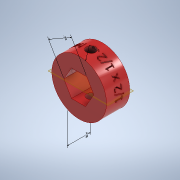
# Autodesk Inventor part: 1_2x1_2-hexBearingSplitA
Saved by Autodesk Inventor 2022.1 (Build 261234000, 234)
## iProperties
Created: 2020-11-08
Part Number: 1_2x1_2-hexBearingSplitA
Material: PC/ABS Plastic
Document SubType Name: Modeling
Designer: robst
Density: 0.357273 g/cm^3
Appearance: Red
Author: robst
Autodesk Inventor part; units mm, degrees
ref_plane "YZ Plane" through (0, 0, 0) normal (1, 0, 0) x (0, 1, 0)
ref_plane "XY Plane" through (0, 0, 0) normal (0, 0, 1) x (1, 0, 0)
sketch "Sketch1" plane through (0, 0, 0) normal (0, 0, 1) x (1, 0, 0)
  line L0 (3.6662, 6.35) -> (7.3323, 0)
  line L1 (7.3323, 0) -> (3.6662, -6.35)
  line L2 (3.6662, -6.35) -> (-3.6662, -6.35)
  line L3 (-3.6662, -6.35) -> (-7.3323, 0)
  line L4 (-7.3323, 0) -> (-3.6662, 6.35)
  line L5 (-3.6662, 6.35) -> (3.6662, 6.35)
  circle A0 centre (0, 0) radius 14.2875
  circle A1 centre (0, 0) radius 7.3323 construction
  dimension "d0" = 12.7
  dimension "d2" = 28.575
  dimension "d3" = 6.9551
  constraints: 12 end point, 3 coincident, 1 centre point, 1 horizontal, 1 horizontal alignment, 15 other
  measures "d0" distance between parallel lines of L2 L5
  measures "d2" diameter of A0
extrude "Extrusion1" add sketch "Sketch1" against normal blind 12.7
thicken "Thicken2" operation add thickness 0.5715 both sides no extend neighbours yes toward (-0.8660254, -0.5, 0) faces at (-4.8882, -4.2333, -4.2333) (-6.1103, 2.1167, -4.2333) (-1.2221, 6.35, -4.2333) (4.8882, 4.2333, -4.2333) (7.8832, 4.3299, 0) (1.2221, -6.35, -4.2333)
ref_plane "Work Plane1" through (0, 14.2875, 0) normal (0, 1, 0) x (-1, 0, 0)
sketch "Sketch2" plane through (0, 14.2875, 0) normal (0, 1, 0) x (-1, 0, 0)
  line L0 (0, -6.9215) -> (-25.4, -6.9215) construction
  line L1 (14.2875, -0.5715) -> (-14.2875, -0.5715) construction
  line L2 (-22.9639, -8.8265) -> (-24.8226, -8.8265)
  line L3 (-24.8226, -8.8265) -> (-24.8226, -8.4375)
  line L4 (-24.8226, -8.4375) -> (-24.131, -8.4375)
  line L5 (-24.131, -8.4375) -> (-24.131, -5.8841)
  line L6 (-24.131, -5.8841) -> (-24.8226, -5.8841)
  line L7 (-24.8226, -5.8841) -> (-24.8226, -5.5352)
  spline S0 degree 2 poles (-24.8226, -5.5352) (-24.4305, -5.5352) (-24.06, -5.3129) (-24.0353, -5.0041) knots 0 0 0 1 2 2 2
  line L8 (-24.0353, -5.0041) -> (-23.6401, -5.0041)
  line L9 (-23.6401, -5.0041) -> (-23.6401, -8.4375)
  line L10 (-23.6401, -8.4375) -> (-22.9639, -8.4375)
  line L11 (-22.9639, -8.4375) -> (-22.9639, -8.8265)
  line L12 (-20.6792, -4.8467) -> (-22.1705, -9.654)
  line L13 (-22.1705, -9.654) -> (-22.6027, -9.654)
  line L14 (-22.6027, -9.654) -> (-21.1176, -4.8467)
  line L15 (-21.1176, -4.8467) -> (-20.6792, -4.8467)
  line L16 (-17.9097, -8.8265) -> (-20.2593, -8.8265)
  line L17 (-20.2593, -8.8265) -> (-20.2593, -8.2862)
  spline S1 degree 2 poles (-20.2593, -8.2862) (-20.0061, -8.0484) (-19.5553, -7.6069) (-19.3392, -7.3692) knots 0 0 0 1 2 2 2
  spline S2 degree 2 poles (-19.3392, -7.3692) (-18.9039, -6.8906) (-18.5858, -6.3163) (-18.5858, -6.0107) knots 0 0 0 1 2 2 2
  spline S3 degree 2 poles (-18.5858, -6.0107) (-18.5858, -5.8501) (-18.6846, -5.6093) (-18.7742, -5.5321) knots 0 0 0 1 2 2 2
  spline S4 degree 2 poles (-18.7742, -5.5321) (-18.8637, -5.4549) (-19.0984, -5.3777) (-19.2404, -5.3777) knots 0 0 0 1 2 2 2
  spline S5 degree 2 poles (-19.2404, -5.3777) (-19.3762, -5.3777) (-19.6541, -5.4457) (-19.7807, -5.4982) knots 0 0 0 1 2 2 2
  spline S6 degree 2 poles (-19.7807, -5.4982) (-19.8888, -5.5414) (-20.0895, -5.6649) (-20.1512, -5.7081) knots 0 0 0 1 2 2 2
  line L18 (-20.1512, -5.7081) -> (-20.179, -5.7081)
  line L19 (-20.179, -5.7081) -> (-20.179, -5.1647)
  spline S7 degree 2 poles (-20.179, -5.1647) (-20.0215, -5.0875) (-19.4565, -4.9362) (-19.2033, -4.9362) knots 0 0 0 1 2 2 2
  spline S8 degree 2 poles (-19.2033, -4.9362) (-18.6692, -4.9362) (-18.0671, -5.5012) (-18.0671, -5.9829) knots 0 0 0 1 2 2 2
  spline S9 degree 2 poles (-18.0671, -5.9829) (-18.0671, -6.2083) (-18.1721, -6.585) (-18.2647, -6.7455) knots 0 0 0 1 2 2 2
  spline S10 degree 2 poles (-18.2647, -6.7455) (-18.3574, -6.9122) (-18.626, -7.2395) (-18.7742, -7.397) knots 0 0 0 1 2 2 2
  spline S11 degree 2 poles (-18.7742, -7.397) (-19.015, -7.6594) (-19.6047, -8.2213) (-19.7807, -8.385) knots 0 0 0 1 2 2 2
  line L20 (-19.7807, -8.385) -> (-17.9097, -8.385)
  line L21 (-17.9097, -8.385) -> (-17.9097, -8.8265)
  line L22 (-13.4729, -8.8265) -> (-14.0626, -8.8265)
  line L23 (-14.0626, -8.8265) -> (-14.7573, -7.752)
  line L24 (-14.7573, -7.752) -> (-15.4705, -8.8265)
  line L25 (-15.4705, -8.8265) -> (-16.017, -8.8265)
  line L26 (-16.017, -8.8265) -> (-15.0259, -7.4093)
  line L27 (-15.0259, -7.4093) -> (-16.0078, -5.9675)
  line L28 (-16.0078, -5.9675) -> (-15.418, -5.9675)
  line L29 (-15.418, -5.9675) -> (-14.7264, -7.0327)
  line L30 (-14.7264, -7.0327) -> (-14.0194, -5.9675)
  line L31 (-14.0194, -5.9675) -> (-13.4729, -5.9675)
  line L32 (-13.4729, -5.9675) -> (-14.4578, -7.3785)
  line L33 (-14.4578, -7.3785) -> (-13.4729, -8.8265)
  line L34 (-9.3758, -8.8265) -> (-11.2345, -8.8265)
  line L35 (-11.2345, -8.8265) -> (-11.2345, -8.4375)
  line L36 (-11.2345, -8.4375) -> (-10.5429, -8.4375)
  line L37 (-10.5429, -8.4375) -> (-10.5429, -5.8841)
  line L38 (-10.5429, -5.8841) -> (-11.2345, -5.8841)
  line L39 (-11.2345, -5.8841) -> (-11.2345, -5.5352)
  spline S12 degree 2 poles (-11.2345, -5.5352) (-10.8423, -5.5352) (-10.4718, -5.3129) (-10.4471, -5.0041) knots 0 0 0 1 2 2 2
  line L40 (-10.4471, -5.0041) -> (-10.0519, -5.0041)
  line L41 (-10.0519, -5.0041) -> (-10.0519, -8.4375)
  line L42 (-10.0519, -8.4375) -> (-9.3758, -8.4375)
  line L43 (-9.3758, -8.4375) -> (-9.3758, -8.8265)
  line L44 (-7.091, -4.8467) -> (-8.5823, -9.654)
  line L45 (-8.5823, -9.654) -> (-9.0145, -9.654)
  line L46 (-9.0145, -9.654) -> (-7.5294, -4.8467)
  line L47 (-7.5294, -4.8467) -> (-7.091, -4.8467)
  line L48 (-4.3215, -8.8265) -> (-6.6711, -8.8265)
  line L49 (-6.6711, -8.8265) -> (-6.6711, -8.2862)
  spline S13 degree 2 poles (-6.6711, -8.2862) (-6.4179, -8.0484) (-5.9671, -7.6069) (-5.751, -7.3692) knots 0 0 0 1 2 2 2
  spline S14 degree 2 poles (-5.751, -7.3692) (-5.3157, -6.8906) (-4.9977, -6.3163) (-4.9977, -6.0107) knots 0 0 0 1 2 2 2
  spline S15 degree 2 poles (-4.9977, -6.0107) (-4.9977, -5.8501) (-5.0965, -5.6093) (-5.186, -5.5321) knots 0 0 0 1 2 2 2
  spline S16 degree 2 poles (-5.186, -5.5321) (-5.2755, -5.4549) (-5.5102, -5.3777) (-5.6522, -5.3777) knots 0 0 0 1 2 2 2
  spline S17 degree 2 poles (-5.6522, -5.3777) (-5.7881, -5.3777) (-6.0659, -5.4457) (-6.1925, -5.4982) knots 0 0 0 1 2 2 2
  spline S18 degree 2 poles (-6.1925, -5.4982) (-6.3006, -5.5414) (-6.5013, -5.6649) (-6.563, -5.7081) knots 0 0 0 1 2 2 2
  line L50 (-6.563, -5.7081) -> (-6.5908, -5.7081)
  line L51 (-6.5908, -5.7081) -> (-6.5908, -5.1647)
  spline S19 degree 2 poles (-6.5908, -5.1647) (-6.4334, -5.0875) (-5.8683, -4.9362) (-5.6152, -4.9362) knots 0 0 0 1 2 2 2
  spline S20 degree 2 poles (-5.6152, -4.9362) (-5.081, -4.9362) (-4.479, -5.5012) (-4.479, -5.9829) knots 0 0 0 1 2 2 2
  spline S21 degree 2 poles (-4.479, -5.9829) (-4.479, -6.2083) (-4.5839, -6.585) (-4.6766, -6.7455) knots 0 0 0 1 2 2 2
  spline S22 degree 2 poles (-4.6766, -6.7455) (-4.7692, -6.9122) (-5.0378, -7.2395) (-5.186, -7.397) knots 0 0 0 1 2 2 2
  spline S23 degree 2 poles (-5.186, -7.397) (-5.4268, -7.6594) (-6.0165, -8.2213) (-6.1925, -8.385) knots 0 0 0 1 2 2 2
  line L52 (-6.1925, -8.385) -> (-4.3215, -8.385)
  line L53 (-4.3215, -8.385) -> (-4.3215, -8.8265)
  line L54 (6.6855, -8.8265) -> (6.2039, -8.8265)
  line L55 (6.2039, -8.8265) -> (6.2039, -7.1963)
  spline S24 degree 2 poles (6.2039, -7.1963) (6.2039, -6.9987) (6.1668, -6.6591) (6.1112, -6.5572) knots 0 0 0 1 2 2 2
  spline S25 degree 2 poles (6.1112, -6.5572) (6.0526, -6.4491) (5.8426, -6.3441) (5.6635, -6.3441) knots 0 0 0 1 2 2 2
  spline S26 degree 2 poles (5.6635, -6.3441) (5.4845, -6.3441) (5.1047, -6.5356) (4.9225, -6.6899) knots 0 0 0 1 2 2 2
  line L56 (4.9225, -6.6899) -> (4.9225, -8.8265)
  line L57 (4.9225, -8.8265) -> (4.4409, -8.8265)
  line L58 (4.4409, -8.8265) -> (4.4409, -4.8467)
  line L59 (4.4409, -4.8467) -> (4.9225, -4.8467)
  line L60 (4.9225, -4.8467) -> (4.9225, -6.2855)
  spline S27 degree 2 poles (4.9225, -6.2855) (5.1387, -6.091) (5.5555, -5.8872) (5.7901, -5.8872) knots 0 0 0 1 2 2 2
  spline S28 degree 2 poles (5.7901, -5.8872) (6.21, -5.8872) (6.6855, -6.4429) (6.6855, -6.9709) knots 0 0 0 1 2 2 2
  line L61 (6.6855, -6.9709) -> (6.6855, -8.8265)
  spline S29 degree 2 poles (8.6029, -8.8913) (7.9174, -8.8913) (7.1641, -8.1225) (7.1641, -7.4124) knots 0 0 0 1 2 2 2
  spline S30 degree 2 poles (7.1641, -7.4124) (7.1641, -6.7146) (7.8958, -5.8872) (8.4855, -5.8872) knots 0 0 0 1 2 2 2
  spline S31 degree 2 poles (8.4855, -5.8872) (8.7511, -5.8872) (9.1617, -6.0416) (9.313, -6.2052) knots 0 0 0 1 2 2 2
  spline S32 degree 2 poles (9.313, -6.2052) (9.4674, -6.3688) (9.631, -6.8412) (9.631, -7.1839) knots 0 0 0 1 2 2 2
  line L62 (9.631, -7.1839) -> (9.631, -7.4464)
  line L63 (9.631, -7.4464) -> (7.6519, -7.4464)
  spline S33 degree 2 poles (7.6519, -7.4464) (7.6519, -7.9435) (8.1521, -8.4714) (8.5967, -8.4714) knots 0 0 0 1 2 2 2
  spline S34 degree 2 poles (8.5967, -8.4714) (8.7541, -8.4714) (9.0598, -8.4004) (9.1833, -8.3448) knots 0 0 0 1 2 2 2
  spline S35 degree 2 poles (9.1833, -8.3448) (9.313, -8.2831) (9.4921, -8.175) (9.5507, -8.1256) knots 0 0 0 1 2 2 2
  line L64 (9.5507, -8.1256) -> (9.5785, -8.1256)
  line L65 (9.5785, -8.1256) -> (9.5785, -8.6505)
  spline S36 degree 2 poles (9.5785, -8.6505) (9.4952, -8.6845) (9.242, -8.7833) (9.1432, -8.8111) knots 0 0 0 1 2 2 2
  spline S37 degree 2 poles (9.1432, -8.8111) (9.0042, -8.8512) (8.7758, -8.8913) (8.6029, -8.8913) knots 0 0 0 1 2 2 2
  spline S38 degree 2 poles (9.1617, -7.079) (9.1555, -6.8844) (9.0753, -6.6004) (8.9981, -6.5047) knots 0 0 0 1 2 2 2
  spline S39 degree 2 poles (8.9981, -6.5047) (8.9147, -6.3966) (8.6523, -6.2824) (8.4577, -6.2824) knots 0 0 0 1 2 2 2
  spline S40 degree 2 poles (8.4577, -6.2824) (8.2663, -6.2824) (7.9977, -6.3966) (7.8866, -6.5078) knots 0 0 0 1 2 2 2
  spline S41 degree 2 poles (7.8866, -6.5078) (7.7785, -6.622) (7.6673, -6.8968) (7.6519, -7.079) knots 0 0 0 1 2 2 2
  line L66 (7.6519, -7.079) -> (9.1617, -7.079)
  line L67 (12.3388, -8.8265) -> (11.749, -8.8265)
  line L68 (11.749, -8.8265) -> (11.0544, -7.752)
  line L69 (11.0544, -7.752) -> (10.3411, -8.8265)
  line L70 (10.3411, -8.8265) -> (9.7946, -8.8265)
  line L71 (9.7946, -8.8265) -> (10.7857, -7.4093)
  line L72 (10.7857, -7.4093) -> (9.8039, -5.9675)
  line L73 (9.8039, -5.9675) -> (10.3936, -5.9675)
  line L74 (10.3936, -5.9675) -> (11.0852, -7.0327)
  line L75 (11.0852, -7.0327) -> (11.7923, -5.9675)
  line L76 (11.7923, -5.9675) -> (12.3388, -5.9675)
  line L77 (12.3388, -5.9675) -> (11.3538, -7.3785)
  line L78 (11.3538, -7.3785) -> (12.3388, -8.8265)
  spline S42 degree 2 poles (16.7447, -7.3507) (16.7447, -8.0515) (16.0654, -8.9068) (15.5529, -8.9068) knots 0 0 0 1 2 2 2
  spline S43 degree 2 poles (15.5529, -8.9068) (15.3213, -8.9068) (14.9909, -8.7925) (14.8304, -8.6937) knots 0 0 0 1 2 2 2
  line L79 (14.8304, -8.6937) -> (14.7995, -8.8265)
  line L80 (14.7995, -8.8265) -> (14.3487, -8.8265)
  line L81 (14.3487, -8.8265) -> (14.3487, -4.8467)
  line L82 (14.3487, -4.8467) -> (14.8304, -4.8467)
  line L83 (14.8304, -4.8467) -> (14.8304, -6.2669)
  spline S44 degree 2 poles (14.8304, -6.2669) (15.0126, -6.1033) (15.4355, -5.8872) (15.7042, -5.8872) knots 0 0 0 1 2 2 2
  spline S45 degree 2 poles (15.7042, -5.8872) (16.1889, -5.8872) (16.7447, -6.6621) (16.7447, -7.3507) knots 0 0 0 1 2 2 2
  spline S46 degree 2 poles (16.2476, -7.3877) (16.2476, -6.8752) (15.9357, -6.3441) (15.5899, -6.3441) knots 0 0 0 1 2 2 2
  spline S47 degree 2 poles (15.5899, -6.3441) (15.3954, -6.3441) (14.994, -6.5294) (14.8304, -6.6714) knots 0 0 0 1 2 2 2
  line L84 (14.8304, -6.6714) -> (14.8304, -8.3109)
  spline S48 degree 2 poles (14.8304, -8.3109) (15.0126, -8.4004) (15.2935, -8.4745) (15.4602, -8.4745) knots 0 0 0 1 2 2 2
  spline S49 degree 2 poles (15.4602, -8.4745) (15.8277, -8.4745) (16.2476, -7.9527) (16.2476, -7.3877) knots 0 0 0 1 2 2 2
  line L85 (19.4678, -8.8265) -> (18.9862, -8.8265)
  line L86 (18.9862, -8.8265) -> (18.9862, -8.5116)
  spline S50 degree 2 poles (18.9862, -8.5116) (18.7639, -8.7061) (18.3656, -8.9068) (18.1186, -8.9068) knots 0 0 0 1 2 2 2
  spline S51 degree 2 poles (18.1186, -8.9068) (17.9333, -8.9068) (17.603, -8.7833) (17.4826, -8.6505) knots 0 0 0 1 2 2 2
  spline S52 degree 2 poles (17.4826, -8.6505) (17.3591, -8.5177) (17.2232, -8.1133) (17.2232, -7.8231) knots 0 0 0 1 2 2 2
  line L87 (17.2232, -7.8231) -> (17.2232, -5.9675)
  line L88 (17.2232, -5.9675) -> (17.7049, -5.9675)
  line L89 (17.7049, -5.9675) -> (17.7049, -7.5977)
  spline S53 degree 2 poles (17.7049, -7.5977) (17.7049, -7.8261) (17.7388, -8.1256) (17.7975, -8.2368) knots 0 0 0 1 2 2 2
  spline S54 degree 2 poles (17.7975, -8.2368) (17.8562, -8.3479) (18.0568, -8.4498) (18.2452, -8.4498) knots 0 0 0 1 2 2 2
  spline S55 degree 2 poles (18.2452, -8.4498) (18.4212, -8.4498) (18.8195, -8.2491) (18.9862, -8.104) knots 0 0 0 1 2 2 2
  line L90 (18.9862, -8.104) -> (18.9862, -5.9675)
  line L91 (18.9862, -5.9675) -> (19.4678, -5.9675)
  line L92 (19.4678, -5.9675) -> (19.4678, -8.8265)
  spline S56 degree 2 poles (20.9375, -8.8944) (20.6504, -8.8944) (20.1533, -8.74) (19.9896, -8.6536) knots 0 0 0 1 2 2 2
  line L93 (19.9896, -8.6536) -> (19.9896, -8.1133)
  line L94 (19.9896, -8.1133) -> (20.0143, -8.1133)
  spline S57 degree 2 poles (20.0143, -8.1133) (20.0761, -8.1627) (20.2428, -8.28) (20.3818, -8.3448) knots 0 0 0 1 2 2 2
  spline S58 degree 2 poles (20.3818, -8.3448) (20.5022, -8.4035) (20.7986, -8.49) (20.956, -8.49) knots 0 0 0 1 2 2 2
  spline S59 degree 2 poles (20.956, -8.49) (21.0703, -8.49) (21.3327, -8.4375) (21.3945, -8.3942) knots 0 0 0 1 2 2 2
  spline S60 degree 2 poles (21.3945, -8.3942) (21.484, -8.3356) (21.5643, -8.2028) (21.5643, -8.067) knots 0 0 0 1 2 2 2
  spline S61 degree 2 poles (21.5643, -8.067) (21.5643, -7.8972) (21.379, -7.7212) (21.1413, -7.6625) knots 0 0 0 1 2 2 2
  spline S62 degree 2 poles (21.1413, -7.6625) (21.0487, -7.6409) (20.7523, -7.5791) (20.6257, -7.5452) knots 0 0 0 1 2 2 2
  spline S63 degree 2 poles (20.6257, -7.5452) (20.2984, -7.4495) (20.002, -7.0543) (20.002, -6.7733) knots 0 0 0 1 2 2 2
  spline S64 degree 2 poles (20.002, -6.7733) (20.002, -6.3843) (20.5855, -5.8995) (21.0672, -5.8995) knots 0 0 0 1 2 2 2
  spline S65 degree 2 poles (21.0672, -5.8995) (21.3049, -5.8995) (21.7866, -6.0169) (21.9502, -6.1064) knots 0 0 0 1 2 2 2
  line L95 (21.9502, -6.1064) -> (21.9502, -6.622)
  line L96 (21.9502, -6.622) -> (21.9255, -6.622)
  spline S66 degree 2 poles (21.9255, -6.622) (21.7403, -6.4738) (21.2895, -6.304) (21.0579, -6.304) knots 0 0 0 1 2 2 2
  spline S67 degree 2 poles (21.0579, -6.304) (20.8202, -6.304) (20.4929, -6.5047) (20.4929, -6.7054) knots 0 0 0 1 2 2 2
  spline S68 degree 2 poles (20.4929, -6.7054) (20.4929, -6.8875) (20.6874, -7.0635) (20.9035, -7.1191) knots 0 0 0 1 2 2 2
  spline S69 degree 2 poles (20.9035, -7.1191) (21.0085, -7.1469) (21.274, -7.2025) (21.4192, -7.2364) knots 0 0 0 1 2 2 2
  spline S70 degree 2 poles (21.4192, -7.2364) (21.7341, -7.3167) (22.0552, -7.6841) (22.0552, -8.0021) knots 0 0 0 1 2 2 2
  spline S71 degree 2 poles (22.0552, -8.0021) (22.0552, -8.1874) (21.9101, -8.5147) (21.768, -8.6351) knots 0 0 0 1 2 2 2
  spline S72 degree 2 poles (21.768, -8.6351) (21.6168, -8.7617) (21.2308, -8.8944) (20.9375, -8.8944) knots 0 0 0 1 2 2 2
  line L97 (24.7475, -8.8265) -> (24.2659, -8.8265)
  line L98 (24.2659, -8.8265) -> (24.2659, -7.1963)
  spline S73 degree 2 poles (24.2659, -7.1963) (24.2659, -6.9987) (24.2288, -6.6591) (24.1732, -6.5572) knots 0 0 0 1 2 2 2
  spline S74 degree 2 poles (24.1732, -6.5572) (24.1146, -6.4491) (23.9046, -6.3441) (23.7255, -6.3441) knots 0 0 0 1 2 2 2
  spline S75 degree 2 poles (23.7255, -6.3441) (23.5465, -6.3441) (23.1667, -6.5356) (22.9845, -6.6899) knots 0 0 0 1 2 2 2
  line L99 (22.9845, -6.6899) -> (22.9845, -8.8265)
  line L100 (22.9845, -8.8265) -> (22.5029, -8.8265)
  line L101 (22.5029, -8.8265) -> (22.5029, -4.8467)
  line L102 (22.5029, -4.8467) -> (22.9845, -4.8467)
  line L103 (22.9845, -4.8467) -> (22.9845, -6.2855)
  spline S76 degree 2 poles (22.9845, -6.2855) (23.2007, -6.091) (23.6175, -5.8872) (23.8521, -5.8872) knots 0 0 0 1 2 2 2
  spline S77 degree 2 poles (23.8521, -5.8872) (24.272, -5.8872) (24.7475, -6.4429) (24.7475, -6.9709) knots 0 0 0 1 2 2 2
  line L104 (24.7475, -6.9709) -> (24.7475, -8.8265)
  line L105 (25.9146, -8.8265) -> (25.4329, -8.8265)
  line L106 (25.4329, -8.8265) -> (25.4329, -5.9675)
  line L107 (25.4329, -5.9675) -> (25.9146, -5.9675)
  line L108 (25.9146, -5.9675) -> (25.9146, -8.8265)
  line L109 (25.9486, -5.492) -> (25.4021, -5.492)
  line L110 (25.4021, -5.492) -> (25.4021, -4.9918)
  line L111 (25.4021, -4.9918) -> (25.9486, -4.9918)
  line L112 (25.9486, -4.9918) -> (25.9486, -5.492)
  line L113 (28.8663, -8.8265) -> (28.3846, -8.8265)
  line L114 (28.3846, -8.8265) -> (28.3846, -7.1963)
  spline S78 degree 2 poles (28.3846, -7.1963) (28.3846, -6.9987) (28.3476, -6.6591) (28.292, -6.5572) knots 0 0 0 1 2 2 2
  spline S79 degree 2 poles (28.292, -6.5572) (28.2333, -6.4491) (28.0234, -6.3441) (27.8443, -6.3441) knots 0 0 0 1 2 2 2
  spline S80 degree 2 poles (27.8443, -6.3441) (27.6652, -6.3441) (27.2854, -6.5356) (27.1033, -6.6899) knots 0 0 0 1 2 2 2
  line L115 (27.1033, -6.6899) -> (27.1033, -8.8265)
  line L116 (27.1033, -8.8265) -> (26.6216, -8.8265)
  line L117 (26.6216, -8.8265) -> (26.6216, -5.9675)
  line L118 (26.6216, -5.9675) -> (27.1033, -5.9675)
  line L119 (27.1033, -5.9675) -> (27.1033, -6.2855)
  spline S81 degree 2 poles (27.1033, -6.2855) (27.3194, -6.091) (27.7362, -5.8872) (27.9709, -5.8872) knots 0 0 0 1 2 2 2
  spline S82 degree 2 poles (27.9709, -5.8872) (28.3908, -5.8872) (28.8663, -6.4429) (28.8663, -6.9709) knots 0 0 0 1 2 2 2
  line L120 (28.8663, -6.9709) -> (28.8663, -8.8265)
  spline S83 degree 2 poles (29.6443, -9.2835) (29.6937, -9.3051) (29.8821, -9.373) (30.0025, -9.4008) knots 0 0 0 1 2 2 2
  spline S84 degree 2 poles (30.0025, -9.4008) (30.1352, -9.4347) (30.3606, -9.4749) (30.4934, -9.4749) knots 0 0 0 1 2 2 2
  spline S85 degree 2 poles (30.4934, -9.4749) (30.7157, -9.4749) (31.0244, -9.3576) (31.1109, -9.2526) knots 0 0 0 1 2 2 2
  spline S86 degree 2 poles (31.1109, -9.2526) (31.1942, -9.1476) (31.2591, -8.8728) (31.2591, -8.6968) knots 0 0 0 1 2 2 2
  line L121 (31.2591, -8.6968) -> (31.2591, -8.4467)
  spline S87 degree 2 poles (31.2591, -8.4467) (31.0646, -8.6165) (30.691, -8.7771) (30.41, -8.7771) knots 0 0 0 1 2 2 2
  spline S88 degree 2 poles (30.41, -8.7771) (29.9222, -8.7771) (29.3448, -8.0515) (29.3448, -7.3692) knots 0 0 0 1 2 2 2
  spline S89 degree 2 poles (29.3448, -7.3692) (29.3448, -7.0141) (29.5455, -6.4645) (29.7122, -6.27) knots 0 0 0 1 2 2 2
  spline S90 degree 2 poles (29.7122, -6.27) (29.8728, -6.0879) (30.3143, -5.8872) (30.549, -5.8872) knots 0 0 0 1 2 2 2
  spline S91 degree 2 poles (30.549, -5.8872) (30.7713, -5.8872) (31.0954, -5.9922) (31.2591, -6.0879) knots 0 0 0 1 2 2 2
  line L122 (31.2591, -6.0879) -> (31.2869, -5.9675)
  line L123 (31.2869, -5.9675) -> (31.7407, -5.9675)
  line L124 (31.7407, -5.9675) -> (31.7407, -8.4992)
  spline S92 degree 2 poles (31.7407, -8.4992) (31.7407, -9.2279) (31.1078, -9.9071) (30.4563, -9.9071) knots 0 0 0 1 2 2 2
  spline S93 degree 2 poles (30.4563, -9.9071) (30.2464, -9.9071) (29.808, -9.8392) (29.6196, -9.7836) knots 0 0 0 1 2 2 2
  line L125 (29.6196, -9.7836) -> (29.6196, -9.2835)
  line L126 (29.6196, -9.2835) -> (29.6443, -9.2835)
  line L127 (31.2591, -8.0515) -> (31.2591, -6.48)
  spline S94 degree 2 poles (31.2591, -6.48) (31.08, -6.3935) (30.7774, -6.3194) (30.6261, -6.3194) knots 0 0 0 1 2 2 2
  spline S95 degree 2 poles (30.6261, -6.3194) (30.2618, -6.3194) (29.8419, -6.8567) (29.8419, -7.3599) knots 0 0 0 1 2 2 2
  spline S96 degree 2 poles (29.8419, -7.3599) (29.8419, -7.8354) (30.1599, -8.3325) (30.5181, -8.3325) knots 0 0 0 1 2 2 2
  spline S97 degree 2 poles (30.5181, -8.3325) (30.7064, -8.3325) (31.1016, -8.1843) (31.2591, -8.0515) knots 0 0 0 1 2 2 2
  spline S98 degree 2 poles (36.4708, -7.3198) (36.4708, -8.0361) (35.7885, -8.8821) (35.2667, -8.8821) knots 0 0 0 1 2 2 2
  spline S99 degree 2 poles (35.2667, -8.8821) (35.0536, -8.8821) (34.7264, -8.7833) (34.5566, -8.6814) knots 0 0 0 1 2 2 2
  line L128 (34.5566, -8.6814) -> (34.5566, -9.8793)
  line L129 (34.5566, -9.8793) -> (34.0749, -9.8793)
  line L130 (34.0749, -9.8793) -> (34.0749, -5.9675)
  line L131 (34.0749, -5.9675) -> (34.5566, -5.9675)
  line L132 (34.5566, -5.9675) -> (34.5566, -6.2669)
  spline S100 degree 2 poles (34.5566, -6.2669) (34.7356, -6.1033) (35.1741, -5.8872) (35.4303, -5.8872) knots 0 0 0 1 2 2 2
  spline S101 degree 2 poles (35.4303, -5.8872) (35.9212, -5.8872) (36.4708, -6.6652) (36.4708, -7.3198) knots 0 0 0 1 2 2 2
  spline S102 degree 2 poles (35.9737, -7.3754) (35.9737, -6.8844) (35.6619, -6.3441) (35.313, -6.3441) knots 0 0 0 1 2 2 2
  spline S103 degree 2 poles (35.313, -6.3441) (35.1092, -6.3441) (34.7264, -6.5263) (34.5566, -6.6683) knots 0 0 0 1 2 2 2
  line L133 (34.5566, -6.6683) -> (34.5566, -8.2924)
  spline S104 degree 2 poles (34.5566, -8.2924) (34.7449, -8.3819) (35.0135, -8.4498) (35.1864, -8.4498) knots 0 0 0 1 2 2 2
  spline S105 degree 2 poles (35.1864, -8.4498) (35.56, -8.4498) (35.9737, -7.9002) (35.9737, -7.3754) knots 0 0 0 1 2 2 2
  line L134 (39.2156, -5.9675) -> (38.1381, -8.8265)
  line L135 (38.1381, -8.8265) -> (37.7058, -8.8265)
  line L136 (37.7058, -8.8265) -> (36.6375, -5.9675)
  line L137 (36.6375, -5.9675) -> (37.1593, -5.9675)
  line L138 (37.1593, -5.9675) -> (37.9405, -8.1689)
  line L139 (37.9405, -8.1689) -> (38.7154, -5.9675)
  line L140 (38.7154, -5.9675) -> (39.2156, -5.9675)
  spline S106 degree 2 poles (41.8802, -6.9215) (41.8802, -7.9466) (41.2843, -8.9068) (40.6637, -8.9068) knots 0 0 0 1 2 2 2
  spline S107 degree 2 poles (40.6637, -8.9068) (40.0338, -8.9068) (39.4441, -7.928) (39.4441, -6.9246) knots 0 0 0 1 2 2 2
  spline S108 degree 2 poles (39.4441, -6.9246) (39.4441, -5.8934) (40.04, -4.9393) (40.6637, -4.9393) knots 0 0 0 1 2 2 2
  spline S109 degree 2 poles (40.6637, -4.9393) (41.2904, -4.9393) (41.8802, -5.9273) (41.8802, -6.9215) knots 0 0 0 1 2 2 2
  spline S110 degree 2 poles (41.2256, -8.0824) (41.2997, -7.8941) (41.3615, -7.3136) (41.3615, -6.9215) knots 0 0 0 1 2 2 2
  spline S111 degree 2 poles (41.3615, -6.9215) (41.3615, -6.5294) (41.2997, -5.952) (41.2225, -5.7575) knots 0 0 0 1 2 2 2
  spline S112 degree 2 poles (41.2225, -5.7575) (41.1453, -5.563) (40.8767, -5.3623) (40.6637, -5.3623) knots 0 0 0 1 2 2 2
  spline S113 degree 2 poles (40.6637, -5.3623) (40.4506, -5.3623) (40.1758, -5.563) (40.0956, -5.7637) knots 0 0 0 1 2 2 2
  spline S114 degree 2 poles (40.0956, -5.7637) (40.0184, -5.9582) (39.9628, -6.551) (39.9628, -6.9246) knots 0 0 0 1 2 2 2
  spline S115 degree 2 poles (39.9628, -6.9246) (39.9628, -7.326) (40.0122, -7.8632) (40.0925, -8.0731) knots 0 0 0 1 2 2 2
  spline S116 degree 2 poles (40.0925, -8.0731) (40.1666, -8.2707) (40.4414, -8.4838) (40.6637, -8.4838) knots 0 0 0 1 2 2 2
  spline S117 degree 2 poles (40.6637, -8.4838) (40.8736, -8.4838) (41.1484, -8.2831) (41.2256, -8.0824) knots 0 0 0 1 2 2 2
  spline S118 degree 2 poles (43.3961, -5.3777) (43.2572, -5.3777) (42.9824, -5.4457) (42.8496, -5.4982) knots 0 0 0 1 2 2 2
  spline S119 degree 2 poles (42.8496, -5.4982) (42.7261, -5.5506) (42.544, -5.6618) (42.473, -5.7112) knots 0 0 0 1 2 2 2
  line L141 (42.473, -5.7112) -> (42.4421, -5.7112)
  line L142 (42.4421, -5.7112) -> (42.4421, -5.1709)
  spline S120 degree 2 poles (42.4421, -5.1709) (42.6088, -5.0813) (43.18, -4.9362) (43.4363, -4.9362) knots 0 0 0 1 2 2 2
  spline S121 degree 2 poles (43.4363, -4.9362) (43.6956, -4.9362) (44.0816, -5.0412) (44.239, -5.1524) knots 0 0 0 1 2 2 2
  spline S122 degree 2 poles (44.239, -5.1524) (44.4057, -5.2728) (44.5786, -5.6217) (44.5786, -5.8563) knots 0 0 0 1 2 2 2
  spline S123 degree 2 poles (44.5786, -5.8563) (44.5786, -6.1712) (44.1649, -6.6467) (43.8747, -6.7085) knots 0 0 0 1 2 2 2
  line L143 (43.8747, -6.7085) -> (43.8747, -6.7455)
  spline S124 degree 2 poles (43.8747, -6.7455) (43.9951, -6.7702) (44.2699, -6.8814) (44.3872, -6.9925) knots 0 0 0 1 2 2 2
  spline S125 degree 2 poles (44.3872, -6.9925) (44.5045, -7.1006) (44.6527, -7.4464) (44.6527, -7.6965) knots 0 0 0 1 2 2 2
  spline S126 degree 2 poles (44.6527, -7.6965) (44.6527, -7.9527) (44.4768, -8.3881) (44.3162, -8.5548) knots 0 0 0 1 2 2 2
  spline S127 degree 2 poles (44.3162, -8.5548) (44.1495, -8.7277) (43.6771, -8.9068) (43.3776, -8.9068) knots 0 0 0 1 2 2 2
  spline S128 degree 2 poles (43.3776, -8.9068) (43.0905, -8.9068) (42.5285, -8.7678) (42.3371, -8.6721) knots 0 0 0 1 2 2 2
  line L144 (42.3371, -8.6721) -> (42.3371, -8.1318)
  line L145 (42.3371, -8.1318) -> (42.3742, -8.1318)
  spline S129 degree 2 poles (42.3742, -8.1318) (42.5347, -8.2491) (43.0781, -8.4653) (43.3467, -8.4653) knots 0 0 0 1 2 2 2
  spline S130 degree 2 poles (43.3467, -8.4653) (43.5042, -8.4653) (43.8191, -8.3665) (43.9241, -8.2522) knots 0 0 0 1 2 2 2
  spline S131 degree 2 poles (43.9241, -8.2522) (44.026, -8.138) (44.134, -7.8663) (44.134, -7.6594) knots 0 0 0 1 2 2 2
  spline S132 degree 2 poles (44.134, -7.6594) (44.134, -7.4526) (44.0136, -7.1839) (43.9056, -7.1068) knots 0 0 0 1 2 2 2
  spline S133 degree 2 poles (43.9056, -7.1068) (43.7975, -7.0296) (43.5042, -6.9709) (43.3313, -6.9709) knots 0 0 0 1 2 2 2
  line L146 (43.3313, -6.9709) -> (43.1152, -6.9709)
  line L147 (43.1152, -6.9709) -> (43.1152, -6.5479)
  line L148 (43.1152, -6.5479) -> (43.285, -6.5479)
  spline S134 degree 2 poles (43.285, -6.5479) (43.6277, -6.5479) (44.0599, -6.2206) (44.0599, -5.9088) knots 0 0 0 1 2 2 2
  spline S135 degree 2 poles (44.0599, -5.9088) (44.0599, -5.7637) (43.9488, -5.5568) (43.8593, -5.4951) knots 0 0 0 1 2 2 2
  spline S136 degree 2 poles (43.8593, -5.4951) (43.7635, -5.4302) (43.5289, -5.3777) (43.3961, -5.3777) knots 0 0 0 1 2 2 2
  point P0 (0, 0)
  dimension "d17" = 25.4
  dimension "d18" = 6.35
  constraints: 2 end point, 2 horizontal
  measures "d17" distance of L0.start L0.end
  measures "d18" distance between parallel lines of L0 L1
emboss "Emboss1" sketch "Sketch2" operation cut depth 2.54 direction (0, -1, 0) wrap yes faces at (14.1025, -2.2919, -8.6572)
sketch "Sketch3" plane through (0, 14.2875, 0) normal (0, 1, 0) x (-1, 0, 0)
  line L0 (3.9961, -0.5715) -> (-3.9961, -0.5715) construction
  line L1 (0, -0.5715) -> (0, -12.7) construction
  line L2 (-3.9961, -12.7) -> (3.9961, -12.7) construction
  line L3 (14.2875, -0.5715) -> (-14.2875, -0.5715) projected
  line L4 (-14.2875, -12.7) -> (14.2875, -12.7) projected
  point P0 (0, 0)
  point P1 (0, -6.6357)
  dimension "d28" = 6.0643
  dimension "d29" = 6.0643
  constraints: 3 midpoint, 2 end point
  measures "d28" distance from line of L3 point (0, -6.636)
  measures "d29" distance from line of L4 point (0, -6.636)
hole "Hole1" at (0, 14.2875, -6.6357) direction (0, -1, 0) diameter 4.318 end through all clearance for "Hex Machine Screw" size "#6" standard "Ansi Unified Screw Threads"
sketch "Sketch4" plane through (0, 14.2875, 0) normal (0, 1, 0) x (-1, 0, 0)
  circle A0 centre (0, -6.6357) radius 2.159 projected
  circle A1 centre (0, -6.6357) radius 2.4257
  point P0 (0, 0)
  point P1 (0, -4.445)
  point P2 (2.0138, -5.8255)
  point P3 (2.0136, -7.3829)
  point P4 (1.4342, -8.2178)
  point P5 (-0.3417, -8.7358)
  point P6 (1.6461, -8.001)
  point P7 (1.1668, -8.4205)
  point P8 (1.1668, -4.7875)
  point P9 (1.6461, -5.207)
  point P10 (1.0457, -8.4928)
  point P11 (0.14, -8.7585)
  point P12 (2.125, -6.2226)
  point P13 (-1.8043, -5.4183)
  point P14 (2.1177, -6.2157)
  point P15 (0.209, -4.4869)
  point P16 (2.1177, -6.2157)
  point P17 (0, -8.763)
  dimension "d30" = 4.8514
  constraints: 1 centre point, 1 coincident, 7 other
  measures "d30" diameter of A1
extrude "Extrusion2" cut sketch "Sketch4" against normal blind 5.5524 contours A0 | A1
equation "\"d0\" = hexSize"
equation "\"d2\" = externalDiameter"
equation "\"d4\" = thickness"
equation "\"d8\" = printSpacing"
equation "\"d9\" = printSpacing"
equation "\"hexSize\" = 12.7"
equation "\"externalDiameter\" = 28.575"
equation "\"thickness\" = 12.7"
equation "\"printSpacing\" = 0.5715"
body "Solid1"
